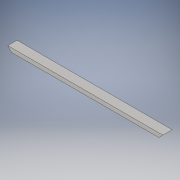
# Autodesk Inventor part: 45 Diagonal Piece
Saved by Autodesk Inventor 2016 (Build 200138000, 138)
## iProperties
Created: 2015-07-05
Part Number: 45 Diagonal Piece
Material: Generic
Document SubType Name: Modeling
Designer: steele
Density: 1 g/cm^3
Appearance: Default
Author: steele
Autodesk Inventor part; units mm, degrees
ref_plane "YZ Plane" through (0, 0, 0) normal (1, 0, 0) x (0, 1, 0)
ref_plane "XZ Plane" through (0, 0, 0) normal (0, 1, 0) x (-1, 0, 0)
ref_plane "XY Plane" through (0, 0, 0) normal (0, 0, 1) x (1, 0, 0)
sketch "Sketch1" plane through (0, 0, 0) normal (0, 0, 1) x (1, 0, 0)
  line L0 (-700.421, -19.05) -> (698.5, -19.05)
  line L1 (736.6, 19.05) -> (-736.6, 19.05)
  line L2 (-736.6, -19.05) -> (736.6, 19.05) construction
  line L3 (736.6, -19.05) -> (-736.6, 19.05) construction
  line L4 (-736.6, 19.05) -> (-700.421, -19.05)
  line L5 (736.6, 19.05) -> (698.5, -19.05)
  point P0 (0, 0)
  dimension "d2" = 45
  dimension "d3" = 45
  dimension "d4" = 38.1
  dimension "length" = 1473.2
  constraints: 12 end point, 2 midpoint, 1 horizontal, 1 parallel
  measures "d2" angle of L4 L3
  measures "d3" angle of L5 L1
  measures "d4" distance between parallel lines of L0 L1
  measures "length" distance of L1.start L1.end
extrude "Extrusion1" add sketch "Sketch1" along normal mid plane 88.9
body "Solid1"
